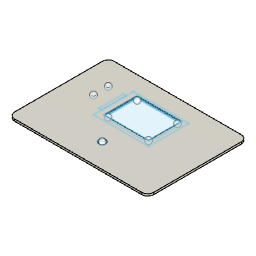
MainUnit_front_panel_V1_0 (Autodesk Fusion 360 design; units mm, degrees)
Autodesk Fusion 360 part; units mm, degrees
sketch "Sketch1" plane through (0, 0, 0) normal (0, 0, 1) x (1, 0, 0)
  line L0 (0, 0) -> (140.94, 0)
  line L1 (140.94, 0) -> (140.94, 100.95)
  line L2 (140.94, 100.95) -> (0, 100.95)
  line L3 (0, 100.95) -> (0, 0)
  dimension "d1" = 140.94
  dimension "d2" = 100.95
  constraint horizontal L0
  constraint vertical L1
  constraint horizontal L2
  constraint vertical L3
  constraint coincident L0.start L3.end
  measures "d1" distance of L0.start L0.end
  measures "d2" distance of L0.start L2.end
extrude "Extrude1" add sketch "Sketch1" along normal blind 2
fillet "Fillet1" radius 6 4 edges at (0, 0, 1) (0, 100.95, 1) (140.94, 100.95, 1) (140.94, 0, 1)
sketch "sketch 796" plane through (0, 0, 2) normal (0, 0, 1) x (-1, 0, 0)
  line L0 (-47.86, -48.85) -> (-92.86, -48.85)
  line L1 (-92.86, -48.85) -> (-92.86, -82.35)
  line L2 (-92.86, -82.35) -> (-47.86, -82.35)
  line L3 (-47.86, -82.35) -> (-47.86, -48.85)
extrude "Extrude2" cut sketch "sketch 796" against normal blind 3
fillet "Fillet2" radius 2 4 edges at (47.86, 82.35, 1) (92.86, 82.35, 1) (92.86, 48.85, 1) (47.86, 48.85, 1)
sketch "sketch 846" plane through (0, 0, 0) normal (0, 0, -1) x (1, 0, 0)
  arc A0 (92.86, -80.35) -> (90.86, -82.35) centre (90.86, -80.35) cw
  line L0 (90.86, -82.35) -> (49.86, -82.35)
  arc A1 (49.86, -82.35) -> (47.86, -80.35) centre (49.86, -80.35) cw
  line L1 (47.86, -80.35) -> (47.86, -50.85)
  arc A2 (47.86, -50.85) -> (49.86, -48.85) centre (49.86, -50.85) cw
  line L2 (49.86, -48.85) -> (90.86, -48.85)
  arc A3 (90.86, -48.85) -> (92.86, -50.85) centre (90.86, -50.85) cw
  line L3 (92.86, -50.85) -> (92.86, -80.35)
  line L4 (96.11, -86.2) -> (40.31, -86.2)
  line L5 (96.11, -45.7) -> (96.11, -86.2)
  line L6 (40.31, -45.7) -> (96.11, -45.7)
  line L7 (40.31, -86.2) -> (40.31, -45.7)
extrude "Extrude3" cut sketch "sketch 846" against normal blind 1
sketch "sketch 818" plane through (0, 0, 2) normal (0, 0, 1) x (-1, 0, 0)
  circle A0 centre (-25, -75.95) radius 1.5
  circle A1 centre (-25, -60.95) radius 1.5
extrude "Extrude4" cut sketch "sketch 818" against normal blind 3
sketch "sketch 834" plane through (0, 0, 2) normal (0, 0, 1) x (-1, 0, 0)
  circle A0 centre (-70.47, -24.425) radius 3.5
extrude "Extrude5" cut sketch "sketch 834" against normal blind 3
sketch "sketch 899" plane through (0, 0, 0) normal (0, 0, -1) x (1, 0, 0)
  line L0 (40.31, -78.95) -> (40.31, -53.95)
  line L1 (40.31, -53.95) -> (37.31, -53.95)
  line L2 (37.31, -53.95) -> (37.31, -78.95)
  line L3 (37.31, -78.95) -> (40.31, -78.95)
extrude "Extrude6" cut sketch "sketch 899" against normal blind 1
